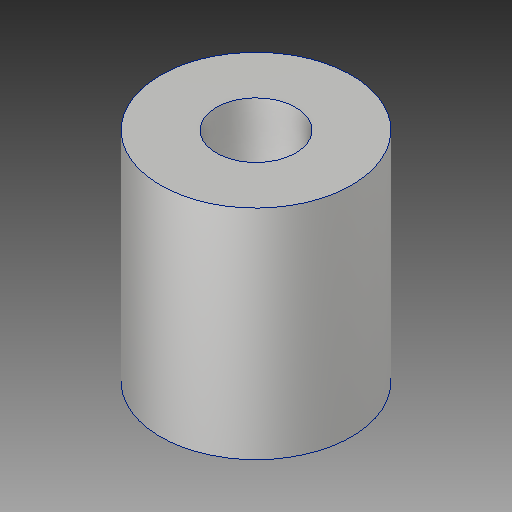
# Autodesk Inventor part: Część2
Saved by Autodesk Inventor 2019.4 (Build 234330000, 330)
## iProperties
Created: 2020-08-31
Part Number: Część2
Material: Aluminium 6061
Document SubType Name: Modeling
Designer: barto
Density: 2.7 g/cm^3
Appearance: Aluminium — płaski
Mass: 48.3467 g
Surface Area: 53.2483 cm^2
Volume: 17.9062 cm^3
Author: barto
Autodesk Inventor part; units mm, degrees
ref_plane "YZ Plane" through (0, 0, 0) normal (1, 0, 0) x (0, 1, 0)
ref_plane "XZ Plane" through (0, 0, 0) normal (0, 1, 0) x (-1, 0, 0)
ref_plane "XY Plane" through (0, 0, 0) normal (0, 0, 1) x (1, 0, 0)
sketch "Szkic1" plane through (0, 0, 0) normal (0, 1, 0) x (-1, 0, 0)
  circle A0 centre (0, 0) radius 6
  circle A1 centre (0, 0) radius 14.4471
  dimension "d0" = 12
  constraints: 2 centre point, 2 coincident
  measures "d0" diameter of A0
extrude "Wyciągnięcie proste1" add sketch "Szkic1" along normal blind 33
